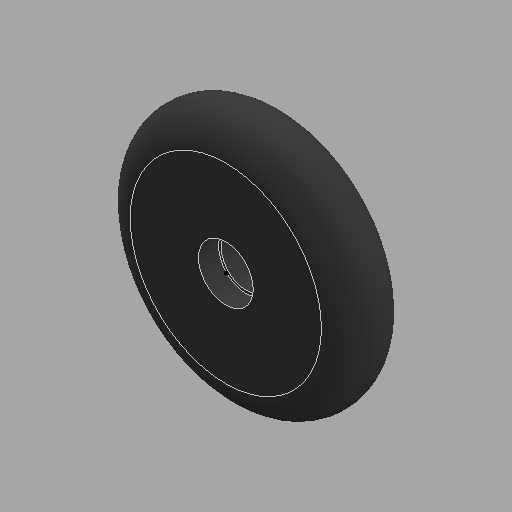
# Autodesk Inventor part: WHEEL
Saved by Autodesk Inventor 2025.2 (Build 292293000, 293)
## iProperties
Created: 2026-06-22
Part Number: WHEEL
Material: Rubber
Document SubType Name: Modeling
Designer: Ben
Density: 0.93 g/cm^3
Appearance: Rubber - Black
Mass: 150.413 g
Surface Area: 208.685 cm^2
Volume: 161.734 cm^3
Author: Ben
Autodesk Inventor part; units mm, degrees
ref_plane "YZ Plane" through (0, 0, 0) normal (1, 0, 0) x (0, 1, 0)
ref_plane "XZ Plane" through (0, 0, 0) normal (0, 1, 0) x (-1, 0, 0)
ref_plane "XY Plane" through (0, 0, 0) normal (0, 0, 1) x (1, 0, 0)
sketch "Sketch1" plane through (0, 0, 0) normal (0, 0, 1) x (1, 0, 0)
  circle A0 centre (0, 0) radius 50
  dimension "d0" = 100
  constraints: 1 centre point, 1 coincident
  measures "d0" diameter of A0
extrude "Extrusion1" add sketch "Sketch1" along normal mid plane 24
fillet "Fillet1" radius 12 2 edges at (-50, 0, 12) (-50, 0, -12)
sketch "Sketch2" plane through (0, 0, 12) normal (0, 0, 1) x (1, 0, 0)
  point P0 (0, 0)
sketch "Sketch3" plane through (0, 0, 12) normal (0, 0, 1) x (1, 0, 0)
  circle A0 centre (0, 0) radius 10.9
  dimension "d4" = 21.8
  constraints: 1 centre point, 1 coincident
  measures "d4" diameter of A0
extrude "Extrusion2" cut sketch "Sketch3" against normal through all
sketch "Sketch4" plane through (0, 0, 0) normal (0, 0, 1) x (1, 0, 0)
  circle A0 centre (0, 0) radius 9.8
  circle A1 centre (0, 0) radius 10.9
  circle A2 centre (0, 0) radius 10.9 projected
  dimension "d7" = 19.6
  constraints: 2 centre point, 2 coincident, 1 concentric
  measures "d7" diameter of A0
extrude "Extrusion4" add sketch "Sketch4" along normal mid plane 8
body "Solid1"
